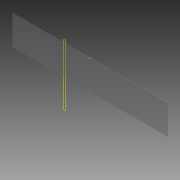
# Autodesk Inventor part: FE-PlayerStationTop
Saved by Autodesk Inventor 2013 (Build 170138000, 138)
## iProperties
Created: 2013-01-14
Part Number: FE-PlayerStationTop
Material: Polycarbonate, Clear
Document SubType Name: Modeling
Designer: Phillip
Density: 1 g/cm^3
Author: Phillip
Autodesk Inventor part; units mm, degrees
ref_plane "YZ Plane" through (0, 0, 0) normal (1, 0, 0) x (0, 1, 0)
ref_plane "XZ Plane" through (0, 0, 0) normal (0, 1, 0) x (-1, 0, 0)
ref_plane "XY Plane" through (0, 0, 0) normal (0, 0, 1) x (1, 0, 0)
ref_plane "Work Plane1" through (0, 0, 0) normal (0, 0, 1) x (1, 0, 0)
sketch "Sketch1" plane through (0, 0, 0) normal (0, 0, 1) x (1, 0, 0)
  line L0 (48214.6435, 12717.2926) -> (46926.203, 12835.6081)
  line L1 (46926.203, 12835.6081) -> (47035.9934, 12184.9022)
  line L2 (44.45, 933.4627) -> (1831.34, 933.4627) projected
  line L3 (44.45, 933.4627) -> (44.45, 889.0127) projected
  line L4 (44.45, 889.0127) -> (1831.34, 889.0127) projected
  line L5 (1831.34, 889.0127) -> (1831.34, 933.4627) projected
  line L6 (44.45, 933.4627) -> (1831.34, 933.4627) projected
  line L7 (-1786.89, 0) -> (-1831.34, 0) projected
  line L8 (-1786.89, 0) -> (-1786.89, 1981.2) projected
  line L9 (-1831.34, 1981.2) -> (-1786.89, 1981.2) projected
  line L10 (-1831.34, 0) -> (-1831.34, 1981.2) projected
  line L11 (-1825.625, 3052.9022) -> (-1825.625, 1986.1022) projected
  line L12 (-1825.625, 1981.2) -> (3698.875, 1981.2)
  line L13 (3698.875, 1981.2) -> (3698.875, 933.4627)
  line L14 (3698.875, 933.4627) -> (-1825.625, 933.4627)
  line L15 (-1825.625, 933.4627) -> (-1825.625, 1981.2)
  line L16 (3698.875, 1986.1022) -> (3698.875, 3052.9022) projected
  point P0 (0, 0)
  constraints: 12 end point, 2 collinear, 2 parallel, 1 horizontal, 1 perpendicular, 1 point on line
extrude "Extrusion1" add sketch "Sketch1" along normal blind 6.35 contours L14 L8 L12 L13 L2 | L14 L15 L9 L8
ref_plane "Work Plane2" through (936.625, 1981.2, 6.35) normal (-1, 0, 0) x (0, -1, 0)
body "Solid1"
